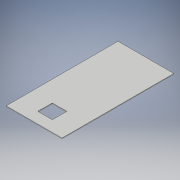
# Autodesk Inventor part: Koffer_dach
Saved by Autodesk Inventor 2018 (Build 220112000, 112)
## iProperties
Created: 2020-03-17
Part Number: Koffer_dach
Material: Generisch
Document SubType Name: Modeling
Designer: wepet
Density: 1 g/cm^3
Appearance: Vorgabe
Author: wepet
Autodesk Inventor part; units mm, degrees
ref_plane "YZ Plane" through (0, 0, 0) normal (1, 0, 0) x (0, 1, 0)
ref_plane "XZ Plane" through (0, 0, 0) normal (0, 1, 0) x (-1, 0, 0)
ref_plane "XY Plane" through (0, 0, 0) normal (0, 0, 1) x (1, 0, 0)
sketch "Skizze1" plane through (0, 0, 0) normal (0, 0, 1) x (1, 0, 0)
  line L0 (-76.5, 0) -> (76.5, 0)
  line L1 (76.5, 0) -> (76.5, 306.5)
  line L2 (76.5, 306.5) -> (-76.5, 306.5)
  line L3 (-76.5, 306.5) -> (-76.5, 0)
  line L4 (75, 306.5) -> (75, 0) construction
  line L5 (-75, 0) -> (-75, 306.5) construction
  line L6 (-76.5, 305) -> (76.5, 305) construction
  point P0 (0, 0)
  point P1 (0, 0)
  point P2 (-75, 305)
  point P3 (75, 305)
  dimension "d2" = 1.5
  dimension "d3" = 1.5
  dimension "d4" = 1.5
  dimension "d5" = 150
  dimension "d6" = 305
  constraints: 14 end point, 10 point on line, 4 perpendicular, 2 parallel, 1 coincident, 1 horizontal, 1 midpoint
  measures "d2" distance between parallel lines of L4 L1
  measures "d3" distance between parallel lines of L3 L5
  measures "d4" distance between parallel lines of L2 L6
  measures "d5" distance between parallel lines of L4 L5
  measures "d6" distance between parallel lines of L0 L6
extrude "Bodenplatte" add sketch "Skizze1" along normal blind 1.8
sketch "Skizze6" plane through (0, 0, 1.8) normal (0, 0, 1) x (1, 0, 0)
  line L0 (-76.5, 306.5) -> (-76.5, 0) construction
  line L1 (-76.5, 0) -> (76.5, 0) construction
  line L2 (76.5, 0) -> (76.5, 306.5) construction
  line L3 (76.5, 306.5) -> (-76.5, 306.5) construction
  line L4 (-76.5, 306.5) -> (-76.5, 0) construction
  line L5 (-18.8, 70) -> (18.8, 70)
  line L6 (20, 68.8) -> (20, 31.2)
  line L7 (18.8, 30) -> (-18.8, 30)
  line L8 (-20, 31.2) -> (-20, 68.8)
  line L9 (0, 0) -> (0, 306.5) construction
  line L10 (76.5, 306.5) -> (-76.5, 306.5) construction
  arc A0 (20, 68.8) -> (18.8, 70) centre (18.8, 68.8) ccw
  arc A1 (-18.8, 70) -> (-20, 68.8) centre (-18.8, 68.8) ccw
  arc A2 (-20, 31.2) -> (-18.8, 30) centre (-18.8, 31.2) ccw
  arc A3 (18.8, 30) -> (20, 31.2) centre (18.8, 31.2) ccw
  point P0 (20, 30)
  point P1 (20, 70)
  point P2 (-20, 30)
  point P3 (0, 30)
  dimension "d18" = 40
  dimension "d19" = 40
  dimension "d20" = 30
  dimension "d21" = 1.2
  dimension "d22" = 1.2
  dimension "d23" = 1.2
  dimension "d24" = 1.2
  constraints: 10 end point, 8 point on circle, 8 tangent, 7 point on line, 4 centre point, 2 midpoint, 2 parallel, 1 horizontal, 1 perpendicular
  measures "d18" distance of point (20, 30) point (-20, 30)
  measures "d19" distance of point (20, 70) point (20, 30)
  measures "d20" distance between parallel lines of L1 L7
  measures "d21" radius of A0
  measures "d22" radius of A1
  measures "d23" radius of A2
  measures "d24" radius of A3
extrude "Extrusion5" cut sketch "Skizze6" against normal up to next
